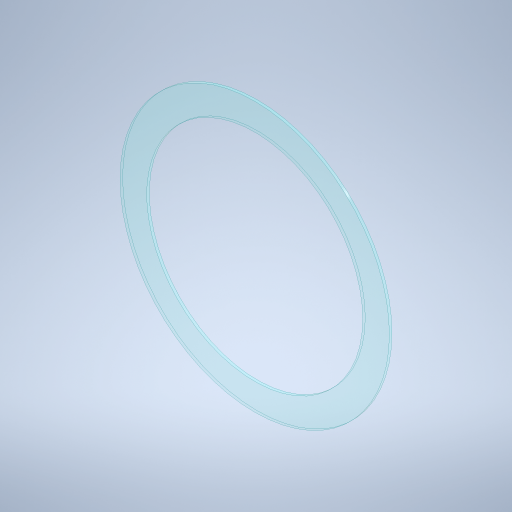
# Autodesk Inventor part: Lid_A
Saved by Autodesk Inventor 2023 (Build 270158000, 158)
## iProperties
Created: 2023-08-16
Part Number: Lid_A
Material: PMMA Plastic
Document SubType Name: Modeling
Designer: Joshua Harper
Density: 1.188 g/cm^3
Appearance: Polycarbonate - Clear
Author: Joshua Harper
Autodesk Inventor part; units mm, degrees
ref_plane "YZ Plane" through (0, 0, 0) normal (1, 0, 0) x (0, 1, 0)
ref_plane "XZ Plane" through (0, 0, 0) normal (0, 1, 0) x (-1, 0, 0)
ref_plane "XY Plane" through (0, 0, 0) normal (0, 0, 1) x (1, 0, 0)
sketch "Sketch1" plane through (0, 0, 0) normal (0, 0, 1) x (1, 0, 0)
  circle A0 centre (0, 0) radius 106
  circle A1 centre (0, 0) radius 85
  dimension "d0" = 170
  dimension "d1" = 212
  constraints: 2 centre point, 2 coincident
  measures "d0" diameter of A1
  measures "d1" diameter of A0
extrude "Extrusion1" add sketch "Sketch1" along normal blind 2
body "Solid1"
